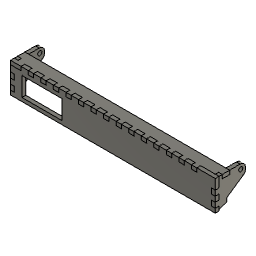
VS-014 v7 (Autodesk Fusion 360 design; units mm, degrees)
Autodesk Fusion 360 part; units mm, degrees
sketch "front" plane through (0, 0, 0) normal (0, 1, 0) x (1, 0, 0)
  line L0 (0, 0) -> (193.6, 0)
  line L1 (193.6, 0) -> (193.6, -28.4)
  line L2 (193.6, -28.4) -> (0, -28.4)
  line L3 (0, -28.4) -> (0, 0)
  line L4 (96.8, 0) -> (96.8, -28.4) construction
  line L5 (0, -28.4) -> (3.6, -28.4)
  line L6 (3.6, -28.4) -> (3.6, 0)
  line L7 (3.6, 0) -> (0, 0)
  line L8 (0, 0) -> (0, -28.4)
  line L9 (190, -28.4) -> (190, 0)
  line L10 (0, -28.4) -> (193.6, -28.4)
  line L11 (193.6, -28.4) -> (193.6, -24.8)
  line L12 (193.6, -24.8) -> (0, -24.8)
  line L13 (0, -24.8) -> (0, -28.4)
  line L14 (10.8793, -21.3552) -> (48.5793, -21.3552)
  line L15 (48.5793, -21.3552) -> (48.5793, -3.3552)
  line L16 (48.5793, -3.3552) -> (10.8793, -3.3552)
  line L17 (10.8793, -3.3552) -> (10.8793, -21.3552)
  line L18 (176.7262, -19.9) -> (180.3262, -19.9) construction
  line L19 (180.3262, -3.6215) -> (176.7262, -3.6215) construction
  line L20 (180.3262, -19.9) -> (183.9262, -19.9)
  line L21 (190, -18.927) -> (193.6, -18.927)
  line L22 (193.6, -18.927) -> (193.6, -13.927)
  line L23 (193.6, -13.927) -> (190, -13.927)
  line L24 (190, -13.927) -> (190, -18.927)
  line L25 (190, -8.927) -> (193.6, -8.927)
  line L26 (193.6, -8.927) -> (193.6, -3.927)
  line L27 (193.6, -3.927) -> (190, -3.927)
  line L28 (190, -3.927) -> (190, -8.927)
  line L29 (0, -15.0692) -> (3.6, -15.0692)
  line L30 (3.6, -15.0692) -> (3.6, -9.4241)
  line L31 (3.6, -9.4241) -> (0, -9.4241)
  line L32 (0, -9.4241) -> (0, -15.0692)
  dimension "d4" = 3.6
  dimension "d5" = 3.6
  dimension "d6" = 28.4
  dimension "d7" = 193.6
  dimension "d8" = 37.7
  dimension "d9" = 18
  dimension "d15" = 3.6
  dimension "d42" = 5
  dimension "d43" = 5
  dimension "d44" = 5
  constraint horizontal L0
  constraint vertical L1
  constraint horizontal L2
  constraint vertical L3
  constraint coincident L0.start L3.end
  constraint midpoint L0 L4.start
  constraint midpoint L2 L4.end
  constraint horizontal L5
  constraint vertical L6
  constraint horizontal L7
  constraint vertical L8
  constraint coincident L0 L6.end
  constraint symmetric L4 L5.end L9.start
  constraint symmetric L4 L6.end L9.end
  constraint horizontal L10
  constraint vertical L11
  constraint horizontal L12
  constraint vertical L13
  constraint coincident L1 L11.end
  constraint horizontal L14
  constraint vertical L15
  constraint horizontal L16
  constraint vertical L17
  constraint horizontal L18
  constraint horizontal L19
  constraint horizontal L20
  constraint horizontal L21
  constraint vertical L22
  constraint horizontal L23
  constraint vertical L24
  constraint coincident L1 L22.end
  constraint coincident L9 L21.start
  constraint horizontal L25
  constraint vertical L26
  constraint horizontal L27
  constraint vertical L28
  constraint coincident L1 L26.end
  constraint coincident L9 L25.start
  constraint horizontal L29
  constraint vertical L30
  constraint horizontal L31
  constraint vertical L32
  constraint coincident L6 L30.end
  constraint coincident L3 L29.start
  measures "d4" distance of L6 L8
  measures "d5" distance of L10 L12
  measures "d6" distance of L0 L2
  measures "d7" distance of L0.start L0.end
  measures "d8" distance of L14.start L14.end
  measures "d9" distance of L14.start L16.end
  measures "d15" distance of L18.start L18.end
  measures "d42" distance of L21 L23
  measures "d43" distance of L25 L27
  measures "d44" distance of L23 L25
sketch "Sketch2" plane through (0, 0, 0) normal (0, 1, 0) x (1, 0, 0)
extrude "Extrude1" add sketch "front" along normal blind 3.6 contours L0 L3 L6 L7 L8 L31 | L0 L6 L9 L12 L24 L28 L30 | L3 L6 L8 L29 L30 L31 L32 | L0 L1 L9 L27 | L3 L6 L8 L12 L29 | L1 L9 L25 L26 L27 L28 | L2 L3 L5 L6 L8 L10 L12 L13 | L1 L9 L23 L25 | L2 L6 L9 L10 L12 | L1 L9 L21 L22 L23 L24 | L1 L9 L12 L21 makes body 1
extrude "Extrude2" add sketch "front" along normal blind 3.6 contours L1 L2 L9 L10 L11 L12 bodies 1
sketch "side" plane through (193.6, 0, 0) normal (1, 0, 0) x (0, 1, 0)
  line L0 (0, 28.4) -> (0, 0)
  line L1 (0, 0) -> (3.6, 0)
  line L2 (3.6, 0) -> (3.6, 28.4)
  line L3 (3.6, 28.4) -> (0, 28.4)
  line L4 (0, 28.4) -> (28.6, 28.4) construction
  line L5 (28.6, 23.4) -> (28.6, 22.0347) construction
  line L6 (28.6, 3.6) -> (0, 3.6) construction
  line L7 (0, 3.6) -> (0, 28.4) construction
  line L8 (0, 28.4) -> (23.6, 28.4)
  line L9 (26.4267, 17.9105) -> (10.8, 7.2)
  line L10 (10.8, 7.2) -> (10.8, 3.6)
  line L11 (10.8, 3.6) -> (0, 0)
  line L12 (0, 0) -> (0, 28.4)
  line L13 (28.6, 28.4) -> (28.6, 19.4)
  circle A0 centre (24.1, 23.9) radius 2
  arc A1 (28.6, 23.4) -> (23.6, 28.4) centre (23.6, 23.4) ccw
  line L14 (0, 0) -> (0, 28.4)
  arc A2 (26.4267, 17.9105) -> (28.6, 22.0347) centre (23.6, 22.0347) ccw
  dimension "d21" = 24.8
  dimension "d22" = 28.6
  dimension "d23" = 9
  dimension "d24" = 3.6
  dimension "d25" = 4
  dimension "d26" = 5
  dimension "d27" = 10.8
  dimension "d28" = 5
  dimension "d29" = 4.5
  dimension "d30" = 4.5
  constraint horizontal L4
  constraint vertical L5
  constraint horizontal L6
  constraint vertical L7
  constraint coincident L0.start L3.end
  constraint coincident L5 L13.end
  constraint coincident L6 L10.end
  constraint perpendicular L6 L10
  constraint coincident L0.end L1.start
  constraint coincident L4.end L8
  constraint coincident L4.end L5
  constraint tangent L8 A1
  constraint tangent L5 A1
  constraint coincident L6.start L5
  constraint coincident L13.end L9
  constraint tangent L5 A2
  constraint tangent L9 A2
  measures "d21" distance of L4.end L6.start
  measures "d22" distance of L0.start L4.end
  measures "d23" distance of L4.end L13.end
  measures "d24" distance of L9.end L10.end
  measures "d25" diameter of A0
  measures "d26" radius of A1
  measures "d27" distance of L10 L14
  measures "d28" radius of A2
  measures "d29" distance of L4 A0.centre
  measures "d30" distance of L13 A0.centre
extrude "Extrude3" add sketch "side" against normal blind 3.6 separate body contours L0 L2 L3 L8 L11 L12 L14 | L2 L8 L9 L10 L11 L13 A1 A2 makes body 2
sketch "top" plane through (0, 0, 28.4) normal (0, 0, 1) x (-1, 0, 0)
  line L0 (0, 0) -> (-193.6, 0)
  line L1 (-193.6, 0) -> (-193.6, -3.6)
  line L2 (-193.6, -3.6) -> (0, -3.6)
  line L3 (0, -3.6) -> (0, 0)
  line L4 (-193.6, -26.4267) -> (-193.6, -28.6)
  line L5 (-190, -28.6) -> (-190, -26.4267)
  line L6 (-193.6, -28.6) -> (-190, -28.6)
  line L7 (-193.6, -10.8) -> (-193.6, 0)
  line L8 (-190, -10.8) -> (-190, 0)
  line L9 (-193.6, -26.4267) -> (-193.6, -10.8)
  line L10 (-190, -26.4267) -> (-190, -10.8)
  line L11 (-193.6, 0) -> (-193.6, -3.6)
  line L12 (0, 0) -> (0, -3.6)
  line L13 (0, 0) -> (-193.6, 0)
  line L14 (-193.6, -3.6) -> (0, -3.6)
  line L15 (-193.6, -13.6) -> (0, -13.6)
  line L16 (-96.8, -13.6) -> (-96.8, 0)
  line L17 (-193.6, -6.6) -> (-190, -6.6)
  line L18 (-190, -3.6) -> (-193.6, -3.6)
  line L19 (-9.8968, -3.6) -> (-9.8968, 0)
  line L20 (-16.7718, 0) -> (-16.7718, -3.6)
  line L21 (-16.7718, -3.6) -> (-21.7718, -3.6)
  line L22 (-21.7718, -3.6) -> (-21.7718, 0)
  line L23 (-28.6468, 0) -> (-28.6468, -3.6)
  line L24 (-28.6468, -3.6) -> (-33.6468, -3.6)
  line L25 (-33.6468, -3.6) -> (-33.6468, 0)
  line L26 (-40.5218, 0) -> (-40.5218, -3.6)
  line L27 (-40.5218, -3.6) -> (-45.5218, -3.6)
  line L28 (-45.5218, -3.6) -> (-45.5218, 0)
  line L29 (-52.3968, 0) -> (-52.3968, -3.6)
  line L30 (-52.3968, -3.6) -> (-57.3968, -3.6)
  line L31 (-57.3968, -3.6) -> (-57.3968, 0)
  line L32 (-64.2718, 0) -> (-64.2718, -3.6)
  line L33 (-64.2718, -3.6) -> (-69.2718, -3.6)
  line L34 (-69.2718, -3.6) -> (-69.2718, 0)
  line L35 (-76.1468, 0) -> (-76.1468, -3.6)
  line L36 (-76.1468, -3.6) -> (-81.1468, -3.6)
  line L37 (-81.1468, -3.6) -> (-81.1468, 0)
  line L38 (-88.0218, 0) -> (-88.0218, -3.6)
  line L39 (-88.0218, -3.6) -> (-93.0218, -3.6)
  line L40 (-93.0218, -3.6) -> (-93.0218, 0)
  line L41 (-99.8968, 0) -> (-99.8968, -3.6)
  line L42 (-99.8968, -3.6) -> (-104.8968, -3.6)
  line L43 (-104.8968, -3.6) -> (-104.8968, 0)
  line L44 (-111.7718, 0) -> (-111.7718, -3.6)
  line L45 (-111.7718, -3.6) -> (-116.7718, -3.6)
  line L46 (-116.7718, -3.6) -> (-116.7718, 0)
  line L47 (-123.6468, 0) -> (-123.6468, -3.6)
  line L48 (-123.6468, -3.6) -> (-128.6468, -3.6)
  line L49 (-128.6468, -3.6) -> (-128.6468, 0)
  line L50 (-135.5218, 0) -> (-135.5218, -3.6)
  line L51 (-135.5218, -3.6) -> (-140.5218, -3.6)
  line L52 (-140.5218, -3.6) -> (-140.5218, 0)
  line L53 (-140.5218, 0) -> (-135.5218, 0)
  line L54 (-147.3968, 0) -> (-147.3968, -3.6)
  line L55 (-147.3968, -3.6) -> (-152.3968, -3.6)
  line L56 (-152.3968, -3.6) -> (-152.3968, 0)
  line L57 (-159.2718, 0) -> (-159.2718, -3.6)
  line L58 (-159.2718, -3.6) -> (-164.2718, -3.6)
  line L59 (-164.2718, -3.6) -> (-164.2718, 0)
  line L60 (-171.1468, 0) -> (-171.1468, -3.6)
  line L61 (-171.1468, -3.6) -> (-176.1468, -3.6)
  line L62 (-176.1468, -3.6) -> (-176.1468, 0)
  line L63 (-193.6, -13.6) -> (-193.6, -6.6)
  line L64 (-190, -6.6) -> (-190, -3.6)
  line L65 (-193.6, -3.6) -> (-193.6, 0)
  line L66 (-188.0218, 0) -> (-193.6, 0)
  line L67 (-176.1468, 0) -> (-183.0218, 0)
  line L68 (-152.3968, 0) -> (-159.2718, 0)
  line L69 (-164.2718, 0) -> (-171.1468, 0)
  line L70 (-140.5218, 0) -> (-147.3968, 0)
  line L71 (-128.6468, 0) -> (-135.5218, 0)
  line L72 (-116.7718, 0) -> (-123.6468, 0)
  line L73 (-104.8968, 0) -> (-111.7718, 0)
  line L74 (-93.0218, 0) -> (-99.8968, 0)
  line L75 (-81.1468, 0) -> (-88.0218, 0)
  line L76 (-57.3968, 0) -> (-64.2718, 0)
  line L77 (-69.2718, 0) -> (-76.1468, 0)
  line L78 (-45.5218, 0) -> (-52.3968, 0)
  line L79 (-33.6468, 0) -> (-40.5218, 0)
  line L80 (-21.7718, 0) -> (-28.6468, 0)
  line L81 (0, 0) -> (-4.8968, 0)
  line L82 (-9.8968, 0) -> (-16.7718, 0)
  line L83 (0, -13.6) -> (0, -6.6)
  line L84 (0, -3.6) -> (0, 0)
  line L85 (-193.6, 0) -> (-193.6, -3.6)
  line L86 (-193.6, -6.6) -> (-193.6, -13.6)
  line L87 (-193.6, -3.6) -> (-4.8968, -3.6) construction
  line L88 (-193.6, 0) -> (-190, 0)
  line L89 (0, -6.6) -> (0, -3.6)
  dimension "d33" = 13.6
  dimension "d34" = 3
  dimension "d35" = 5
  dimension "d47" = 3.6
  constraint horizontal L81
  constraint vertical L85
  constraint horizontal L15
  constraint vertical L83
  constraint coincident L9 L15.start
  constraint coincident L0.start L3.end
  constraint midpoint L15 L16.start
  constraint midpoint L13 L16.end
  constraint horizontal L17
  constraint horizontal L18
  constraint coincident L8 L18.start
  constraint coincident L17.start L85
  constraint vertical L19
  constraint coincident L19.end L81
  constraint coincident L2 L87.end
  constraint symmetric L16 L17.start L83.end
  constraint symmetric L16 L1.end L2.end
  constraint perpendicular L18 L64
  constraint coincident L0.end L1.start
  constraint perpendicular L13 L65
  constraint collinear L66 L81
  constraint collinear L67 L81
  constraint collinear L68 L81
  constraint collinear L68 L69
  constraint collinear L70 L81
  constraint collinear L71 L81
  constraint collinear L72 L81
  constraint collinear L73 L81
  constraint collinear L74 L81
  constraint collinear L75 L81
  constraint collinear L76 L81
  constraint collinear L76 L77
  constraint collinear L78 L81
  constraint collinear L79 L81
  constraint collinear L80 L81
  constraint collinear L81 L82
  constraint collinear L83 L84
  constraint collinear L85 L86
  constraint horizontal L21
  constraint horizontal L24
  constraint collinear L24 L87
  constraint collinear L21 L87
  constraint collinear L27 L87
  constraint collinear L30 L87
  constraint collinear L33 L87
  constraint collinear L36 L87
  constraint collinear L39 L87
  constraint collinear L42 L87
  constraint collinear L45 L87
  constraint collinear L48 L87
  constraint collinear L51 L87
  constraint collinear L55 L87
  constraint collinear L58 L87
  constraint collinear L61 L87
  measures "d33" distance of L0.start L15.end
  measures "d34" distance of L17.end L18.start
  measures "d35" distance of L87.end L19.start
  measures "d47" distance of L75 L87
extrude "Extrude4" add sketch "top" against normal blind 3.6 separate body contours L0 L2 L3 L12 L13 L14 L19 L81 L84 | L2 L14 L15 L16 L21 L24 L27 L30 L33 L36 L39 L83 L89 | L0 L2 L13 L14 L20 L21 L22 | L2 L8 L10 L14 L15 L16 L42 L45 L48 L51 L55 L58 L61 L64 | L0 L2 L13 L14 L23 L24 L25 | L7 L8 L9 L10 L15 L17 L63 L86 | L0 L2 L13 L14 L41 L42 L43 | L0 L2 L13 L14 L38 L39 L40 | L0 L2 L13 L14 L26 L27 L28 | L0 L2 L13 L14 L44 L45 L46 | L0 L2 L13 L14 L35 L36 L37 | L0 L2 L13 L14 L29 L30 L31 | L0 L2 L13 L14 L60 L61 L62 | L0 L2 L13 L14 L47 L48 L49 | L0 L2 L13 L14 L32 L33 L34 | L0 L2 L13 L14 L57 L58 L59 | L0 L2 L13 L14 L50 L51 L52 L53 | L0 L2 L13 L14 L54 L55 L56 makes body 3
combine "Combine2" operation cut target body 1 tool bodies 3 keep tools
extrude "Extrude5" cut sketch "front" along normal blind 3.6 contours L1 L9 L25 L26 L27 L28 | L1 L9 L21 L22 L23 L24 bodies 1
combine "Combine3" operation cut target body 2 tool bodies 1 keep tools
sketch "top DXF" plane through (0, 0, 0) normal (0, 0, 1) x (1, 0, 0)
  line L0 (9.8968, 0) -> (0, 0)
  line L1 (9.8968, 3.6) -> (9.8968, 0)
  line L2 (182.9462, 10.9621) -> (164.0246, 10.9621) construction
  line L3 (164.0246, 10.9621) -> (164.0246, 6.0631) construction
  line L4 (164.0246, 6.0631) -> (182.9462, 6.0631) construction
  line L5 (182.9462, 6.0631) -> (182.9462, 10.9621) construction
  line L6 (0, 13.6) -> (193.6, 13.6)
  line L7 (0, 0) -> (0, 13.6)
  line L8 (16.7718, 3.6) -> (9.8968, 3.6)
  line L9 (16.7718, 0) -> (16.7718, 3.6)
  line L10 (21.7718, 0) -> (16.7718, 0)
  line L11 (21.7718, 3.6) -> (21.7718, 0)
  line L12 (28.6468, 3.6) -> (21.7718, 3.6)
  line L13 (28.6468, 0) -> (28.6468, 3.6)
  line L14 (33.6468, 0) -> (28.6468, 0)
  line L15 (33.6468, 3.6) -> (33.6468, 0)
  line L16 (40.5218, 3.6) -> (33.6468, 3.6)
  line L17 (40.5218, 0) -> (40.5218, 3.6)
  line L18 (45.5218, 0) -> (40.5218, 0)
  line L19 (45.5218, 3.6) -> (45.5218, 0)
  line L20 (52.3968, 3.6) -> (45.5218, 3.6)
  line L21 (52.3968, 0) -> (52.3968, 3.6)
  line L22 (57.3968, 0) -> (52.3968, 0)
  line L23 (57.3968, 3.6) -> (57.3968, 0)
  line L24 (64.2718, 3.6) -> (57.3968, 3.6)
  line L25 (64.2718, 0) -> (64.2718, 3.6)
  line L26 (69.2718, 0) -> (64.2718, 0)
  line L27 (69.2718, 3.6) -> (69.2718, 0)
  line L28 (76.1468, 3.6) -> (69.2718, 3.6)
  line L29 (76.1468, 0) -> (76.1468, 3.6)
  line L30 (81.1468, 0) -> (76.1468, 0)
  line L31 (81.1468, 3.6) -> (81.1468, 0)
  line L32 (88.0218, 3.6) -> (81.1468, 3.6)
  line L33 (88.0218, 0) -> (88.0218, 3.6)
  line L34 (93.0218, 0) -> (88.0218, 0)
  line L35 (93.0218, 3.6) -> (93.0218, 0)
  line L36 (99.8968, 3.6) -> (93.0218, 3.6)
  line L37 (99.8968, 0) -> (99.8968, 3.6)
  line L38 (104.8968, 0) -> (99.8968, 0)
  line L39 (104.8968, 3.6) -> (104.8968, 0)
  line L40 (111.7718, 3.6) -> (104.8968, 3.6)
  line L41 (111.7718, 0) -> (111.7718, 3.6)
  line L42 (116.7718, 0) -> (111.7718, 0)
  line L43 (116.7718, 3.6) -> (116.7718, 0)
  line L44 (123.6468, 3.6) -> (116.7718, 3.6)
  line L45 (123.6468, 0) -> (123.6468, 3.6)
  line L46 (128.6468, 0) -> (123.6468, 0)
  line L47 (128.6468, 3.6) -> (128.6468, 0)
  line L48 (135.5218, 3.6) -> (128.6468, 3.6)
  line L49 (135.5218, 0) -> (135.5218, 3.6)
  line L50 (140.5218, 0) -> (135.5218, 0)
  line L51 (140.5218, 3.6) -> (140.5218, 0)
  line L52 (147.3968, 3.6) -> (140.5218, 3.6)
  line L53 (147.3968, 0) -> (147.3968, 3.6)
  line L54 (152.3968, 0) -> (147.3968, 0)
  line L55 (152.3968, 3.6) -> (152.3968, 0)
  line L56 (159.2718, 3.6) -> (152.3968, 3.6)
  line L57 (159.2718, 0) -> (159.2718, 3.6)
  line L58 (164.2718, 0) -> (159.2718, 0)
  line L59 (164.2718, 3.6) -> (164.2718, 0)
  line L60 (171.1468, 3.6) -> (164.2718, 3.6)
  line L61 (171.1468, 0) -> (171.1468, 3.6)
  line L62 (176.1468, 0) -> (171.1468, 0)
  line L63 (176.1468, 3.6) -> (176.1468, 0)
  line L64 (190, 3.6) -> (176.1468, 3.6)
  line L65 (190, 6.6) -> (190, 3.6)
  line L66 (193.6, 6.6) -> (190, 6.6)
  line L67 (193.6, 13.6) -> (193.6, 6.6)
  dimension "d53" = 3.4
sketch "front dxf" plane through (0, 0, 0) normal (0, -1, 0) x (1, 0, 0)
  line L0 (190, 18.927) -> (193.6, 18.927)
  line L1 (193.6, 18.927) -> (193.6, 28.4)
  line L2 (0, 24.8) -> (0, 0)
  line L3 (0, 0) -> (193.6, 0)
  line L4 (193.6, 0) -> (193.6, 3.927)
  line L5 (193.6, 3.927) -> (190, 3.927)
  line L6 (190, 3.927) -> (190, 8.927)
  line L7 (190, 8.927) -> (193.6, 8.927)
  line L8 (193.6, 8.927) -> (193.6, 13.927)
  line L9 (193.6, 13.927) -> (190, 13.927)
  line L10 (190, 13.927) -> (190, 18.927)
  line L11 (10.8793, 3.3552) -> (10.8793, 21.3552)
  line L12 (10.8793, 21.3552) -> (48.5793, 21.3552)
  line L13 (48.5793, 21.3552) -> (48.5793, 3.3552)
  line L14 (48.5793, 3.3552) -> (10.8793, 3.3552)
  line L15 (190, 13.927) -> (193.6, 13.927)
  line L16 (193.6, 18.927) -> (190, 18.927)
  line L17 (190, 18.927) -> (190, 13.927)
  line L18 (190, 3.927) -> (193.6, 3.927)
  line L19 (193.6, 8.927) -> (190, 8.927)
  line L20 (190, 8.927) -> (190, 3.927)
  line L21 (10.8793, 21.3552) -> (10.8793, 3.3552)
  line L22 (10.8793, 3.3552) -> (48.5793, 3.3552)
  line L23 (48.5793, 3.3552) -> (48.5793, 21.3552)
  line L24 (48.5793, 21.3552) -> (10.8793, 21.3552)
  line L25 (193.6, 0) -> (0, 0)
  line L26 (0, 0) -> (0, 24.8)
  line L27 (193.6, 28.4) -> (176.1468, 28.4)
  line L28 (9.8968, 28.4) -> (9.8968, 24.8)
  line L29 (176.1468, 24.8) -> (171.1468, 24.8)
  line L30 (0, 24.8) -> (9.8968, 24.8)
  line L31 (9.8968, 24.8) -> (9.8968, 28.4)
  line L32 (9.8968, 28.4) -> (16.7718, 28.4)
  line L33 (176.1468, 28.4) -> (176.1468, 24.8)
  line L34 (171.1468, 24.8) -> (171.1468, 28.4)
  line L35 (171.1468, 28.4) -> (164.2718, 28.4)
  line L36 (164.2718, 28.4) -> (164.2718, 24.8)
  line L37 (164.2718, 24.8) -> (159.2718, 24.8)
  line L38 (159.2718, 24.8) -> (159.2718, 28.4)
  line L39 (159.2718, 28.4) -> (152.3968, 28.4)
  line L40 (152.3968, 28.4) -> (152.3968, 24.8)
  line L41 (152.3968, 24.8) -> (147.3968, 24.8)
  line L42 (147.3968, 24.8) -> (147.3968, 28.4)
  line L43 (147.3968, 28.4) -> (140.5218, 28.4)
  line L44 (140.5218, 28.4) -> (140.5218, 24.8)
  line L45 (140.5218, 24.8) -> (135.5218, 24.8)
  line L46 (135.5218, 24.8) -> (135.5218, 28.4)
  line L47 (135.5218, 28.4) -> (128.6468, 28.4)
  line L48 (128.6468, 28.4) -> (128.6468, 24.8)
  line L49 (128.6468, 24.8) -> (123.6468, 24.8)
  line L50 (123.6468, 24.8) -> (123.6468, 28.4)
  line L51 (123.6468, 28.4) -> (116.7718, 28.4)
  line L52 (116.7718, 28.4) -> (116.7718, 24.8)
  line L53 (116.7718, 24.8) -> (111.7718, 24.8)
  line L54 (111.7718, 24.8) -> (111.7718, 28.4)
  line L55 (111.7718, 28.4) -> (104.8968, 28.4)
  line L56 (104.8968, 28.4) -> (104.8968, 24.8)
  line L57 (104.8968, 24.8) -> (99.8968, 24.8)
  line L58 (99.8968, 24.8) -> (99.8968, 28.4)
  line L59 (99.8968, 28.4) -> (93.0218, 28.4)
  line L60 (93.0218, 28.4) -> (93.0218, 24.8)
  line L61 (93.0218, 24.8) -> (88.0218, 24.8)
  line L62 (88.0218, 24.8) -> (88.0218, 28.4)
  line L63 (88.0218, 28.4) -> (81.1468, 28.4)
  line L64 (81.1468, 28.4) -> (81.1468, 24.8)
  line L65 (81.1468, 24.8) -> (76.1468, 24.8)
  line L66 (76.1468, 24.8) -> (76.1468, 28.4)
  line L67 (76.1468, 28.4) -> (69.2718, 28.4)
  line L68 (69.2718, 28.4) -> (69.2718, 24.8)
  line L69 (69.2718, 24.8) -> (64.2718, 24.8)
  line L70 (64.2718, 24.8) -> (64.2718, 28.4)
  line L71 (64.2718, 28.4) -> (57.3968, 28.4)
  line L72 (57.3968, 28.4) -> (57.3968, 24.8)
  line L73 (57.3968, 24.8) -> (52.3968, 24.8)
  line L74 (52.3968, 24.8) -> (52.3968, 28.4)
  line L75 (52.3968, 28.4) -> (45.5218, 28.4)
  line L76 (45.5218, 28.4) -> (45.5218, 24.8)
  line L77 (45.5218, 24.8) -> (40.5218, 24.8)
  line L78 (40.5218, 24.8) -> (40.5218, 28.4)
  line L79 (40.5218, 28.4) -> (33.6468, 28.4)
  line L80 (33.6468, 28.4) -> (33.6468, 24.8)
  line L81 (33.6468, 24.8) -> (28.6468, 24.8)
  line L82 (28.6468, 24.8) -> (28.6468, 28.4)
  line L83 (28.6468, 28.4) -> (21.7718, 28.4)
  line L84 (21.7718, 28.4) -> (21.7718, 24.8)
  line L85 (21.7718, 24.8) -> (16.7718, 24.8)
  line L86 (16.7718, 24.8) -> (16.7718, 28.4)
  line L87 (16.7718, 28.4) -> (9.8968, 28.4)
  line L88 (9.8968, 24.8) -> (0, 24.8)
  line L89 (193.6, 13.927) -> (193.6, 8.927)
  line L90 (193.6, 3.927) -> (193.6, 0)
  line L91 (16.7718, 28.4) -> (16.7718, 24.8)
  line L92 (16.7718, 24.8) -> (21.7718, 24.8)
  line L93 (21.7718, 24.8) -> (21.7718, 28.4)
  line L94 (21.7718, 28.4) -> (28.6468, 28.4)
  line L95 (28.6468, 28.4) -> (28.6468, 24.8)
  line L96 (28.6468, 24.8) -> (33.6468, 24.8)
  line L97 (33.6468, 24.8) -> (33.6468, 28.4)
  line L98 (33.6468, 28.4) -> (40.5218, 28.4)
  line L99 (40.5218, 28.4) -> (40.5218, 24.8)
  line L100 (40.5218, 24.8) -> (45.5218, 24.8)
  line L101 (45.5218, 24.8) -> (45.5218, 28.4)
  line L102 (45.5218, 28.4) -> (52.3968, 28.4)
  line L103 (52.3968, 28.4) -> (52.3968, 24.8)
  line L104 (52.3968, 24.8) -> (57.3968, 24.8)
  line L105 (57.3968, 24.8) -> (57.3968, 28.4)
  line L106 (57.3968, 28.4) -> (64.2718, 28.4)
  line L107 (64.2718, 28.4) -> (64.2718, 24.8)
  line L108 (64.2718, 24.8) -> (69.2718, 24.8)
  line L109 (69.2718, 24.8) -> (69.2718, 28.4)
  line L110 (69.2718, 28.4) -> (76.1468, 28.4)
  line L111 (76.1468, 28.4) -> (76.1468, 24.8)
  line L112 (76.1468, 24.8) -> (81.1468, 24.8)
  line L113 (81.1468, 24.8) -> (81.1468, 28.4)
  line L114 (81.1468, 28.4) -> (88.0218, 28.4)
  line L115 (88.0218, 28.4) -> (88.0218, 24.8)
  line L116 (88.0218, 24.8) -> (93.0218, 24.8)
  line L117 (93.0218, 24.8) -> (93.0218, 28.4)
  line L118 (93.0218, 28.4) -> (99.8968, 28.4)
  line L119 (99.8968, 28.4) -> (99.8968, 24.8)
  line L120 (99.8968, 24.8) -> (104.8968, 24.8)
  line L121 (104.8968, 24.8) -> (104.8968, 28.4)
  line L122 (104.8968, 28.4) -> (111.7718, 28.4)
  line L123 (111.7718, 28.4) -> (111.7718, 24.8)
  line L124 (111.7718, 24.8) -> (116.7718, 24.8)
  line L125 (116.7718, 24.8) -> (116.7718, 28.4)
  line L126 (116.7718, 28.4) -> (123.6468, 28.4)
  line L127 (123.6468, 28.4) -> (123.6468, 24.8)
  line L128 (123.6468, 24.8) -> (128.6468, 24.8)
  line L129 (128.6468, 24.8) -> (128.6468, 28.4)
  line L130 (128.6468, 28.4) -> (135.5218, 28.4)
  line L131 (135.5218, 28.4) -> (135.5218, 24.8)
  line L132 (135.5218, 24.8) -> (140.5218, 24.8)
  line L133 (140.5218, 24.8) -> (140.5218, 28.4)
  line L134 (140.5218, 28.4) -> (147.3968, 28.4)
  line L135 (147.3968, 28.4) -> (147.3968, 24.8)
  line L136 (147.3968, 24.8) -> (152.3968, 24.8)
  line L137 (152.3968, 24.8) -> (152.3968, 28.4)
  line L138 (152.3968, 28.4) -> (159.2718, 28.4)
  line L139 (159.2718, 28.4) -> (159.2718, 24.8)
  line L140 (159.2718, 24.8) -> (164.2718, 24.8)
  line L141 (164.2718, 24.8) -> (164.2718, 28.4)
  line L142 (164.2718, 28.4) -> (171.1468, 28.4)
  line L143 (171.1468, 28.4) -> (171.1468, 24.8)
  line L144 (171.1468, 24.8) -> (176.1468, 24.8)
  line L145 (176.1468, 24.8) -> (176.1468, 28.4)
  line L146 (176.1468, 28.4) -> (193.6, 28.4)
  line L147 (193.6, 28.4) -> (193.6, 18.927)
sketch "side dxf" plane through (193.6, 0, 0) normal (1, 0, 0) x (0, 1, 0)
  line L0 (3.6, 28.4) -> (23.6, 28.4)
  line L1 (0, 8.927) -> (3.6, 8.927)
  line L2 (3.6, 13.927) -> (0, 13.927)
  line L3 (0, 18.927) -> (3.6, 18.927)
  line L4 (3.6, 3.927) -> (0, 3.927)
  line L5 (10.8, 3.6) -> (3.6, 1.2)
  circle A0 centre (24.1, 23.9) radius 2
  arc A1 (28.6, 23.4) -> (23.6, 28.4) centre (23.6, 23.4) ccw
  line L6 (28.6, 23.4) -> (28.6, 22.0347)
  arc A2 (26.4267, 17.9105) -> (28.6, 22.0347) centre (23.6, 22.0347) ccw
  line L7 (26.4267, 17.9105) -> (10.8, 7.2)
  line L8 (10.8, 7.2) -> (10.8, 3.6)
  line L9 (0, 13.927) -> (0, 18.927)
  line L10 (0, 3.927) -> (0, 8.927)
  line L11 (3.6, 8.927) -> (3.6, 13.927)
  line L12 (3.6, 18.927) -> (3.6, 28.4)
  line L13 (3.6, 1.2) -> (3.6, 3.927)
combine "Combine5" operation cut target body 2 tool bodies 3 keep tools
copy_body "CopyPasteBodies2" bodies 2 makes body 4
move_body "Move3" bodies 4 to x (1, 0, 0) y (0, 1, 0) z (0, 0, 1) at (-190, 0, 0)
combine "Combine10" operation cut target body 3 tool bodies 4 keep tools
combine "Combine11" operation cut target body 1 tool bodies 4 keep tools
equation "tapeWidth = ( 95 * 2 ) * 1 mm"
equation "tapeHeight = 24.8 mm"
equation "materialW = 3.6 mm"
equation "d4 = materialW"
equation "d5 = materialW"
equation "d6 = tapeHeight + materialW"
equation "d7 = tapeWidth + materialW"
equation "d15 = materialW"
equation "d17 = materialW"
equation "d19 = materialW"
equation "d21 = tapeHeight"
equation "d22 = tapeHolderDepth + materialW"
equation "d24 = materialW"
equation "d27 = materialW * 3"
equation "d31 = materialW * -1"
equation "d33 = overlapDepth + materialW"
equation "d40 = -materialW"
equation "d45 = materialW"
equation "d47 = materialW"
equation "tapeHolderDepth = 25 mm"
equation "overlapDepth = 10 mm"
named bodies: "front", "side", "top", "side (1)"
